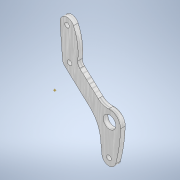
# Autodesk Inventor part: アーノン
Saved by Autodesk Inventor 2022.2 (Build 262287030, 287C)
## iProperties
Created: 2022-01-29
Part Number: アーノン
Material: Aluminum 7075
Document SubType Name: Modeling
Designer: acps
Density: 2.81 g/cm^3
Appearance: Satin - Brushed Heavy
Author: acps
Autodesk Inventor part; units mm, degrees
ref_plane "YZ Plane" through (0, 0, 0) normal (1, 0, 0) x (0, 1, 0)
ref_plane "XZ Plane" through (0, 0, 0) normal (0, 1, 0) x (-1, 0, 0)
ref_plane "XY Plane" through (0, 0, 0) normal (0, 0, 1) x (1, 0, 0)
sketch "Sketch2" plane through (0, 0, 0) normal (0, 0, 1) x (1, 0, 0)
  circle A0 centre (7.8339, 40) radius 4.5
  circle A1 centre (7.8339, 40) radius 1.5
  circle A2 centre (7.8339, 40) radius 5.5 construction
  circle A3 centre (9.4447, 20) radius 5.5 construction
  circle A4 centre (9.4447, 20) radius 4.5
  circle A5 centre (9.4447, 20) radius 1.5
  circle A6 centre (34.6118, -20) radius 5.5 construction
  circle A7 centre (34.6118, -20) radius 4.5
  circle A8 centre (34.6118, -20) radius 1.5
  circle A9 centre (35, 0) radius 9 construction
  line L0 (3.3484, 39.6387) -> (4.9593, 19.6387)
  circle A10 centre (35, 0) radius 7.025
  line L1 (6.404, 16.6828) -> (22.2716, 2.1377)
  line L2 (28.617, -6.3449) -> (29.1733, -11.5166) construction
  circle A11 centre (35, 0) radius 4.025
  line L3 (14.3908, 21.5707) -> (15.9542, 20.1376)
  arc A12 (14.3908, 21.5707) -> (14.4936, 22.1814) centre (-20.0705, 27.6877) ccw
  arc A13 (38.9631, -21.1475) -> (42.0213, -0.228) centre (-51.9292, 2.8233) ccw
  arc A14 (26.106, -1.3771) -> (26.9678, -4.06) centre (35, 0) ccw construction
  arc A15 (14.685, 23.5582) -> (15.9542, 20.1376) centre (18.6571, 23.0862) ccw
  arc A16 (29.1733, -11.5166) -> (22.2716, 2.1377) centre (7.6311, -13.8339) ccw
  line L4 (22.2716, 2.1377) -> (26.106, -1.3771) construction
  arc A17 (26.9678, -4.06) -> (28.617, -6.3449) centre (35, 0) ccw construction
  line L5 (29.1733, -11.5166) -> (30.1377, -20.4813)
  arc A18 (14.4936, 22.1814) -> (11.951, 41.8166) centre (-20.0705, 27.6877) ccw
  line L6 (15.9542, 20.1376) -> (31.3649, 6.0114)
  arc A19 (27.7268, 9.3462) -> (34.4776, 7.0055) centre (33.8083, 15.9806) ccw
  point P0 (0, 0)
  dimension "d17" = 14.05
  dimension "d18" = 8.05
  dimension "d19" = 35
  dimension "d20" = 4
  dimension "d21" = 94
  dimension "d22" = 9
  constraints: 30 point on circle, 26 tangent, 19 centre point, 14 end point, 4 parallel, 2 coincident, 1 concentric, 1 point on line, 12 other
  measures "d17" diameter of A10
  measures "d18" diameter of A11
  measures "d19" radius of A12
  measures "d20" radius of A15
  measures "d21" radius of A13
  measures "d22" radius of A19
extrude "Extrusion2" add sketch "Sketch2" against normal blind 3
body "Solid2"
